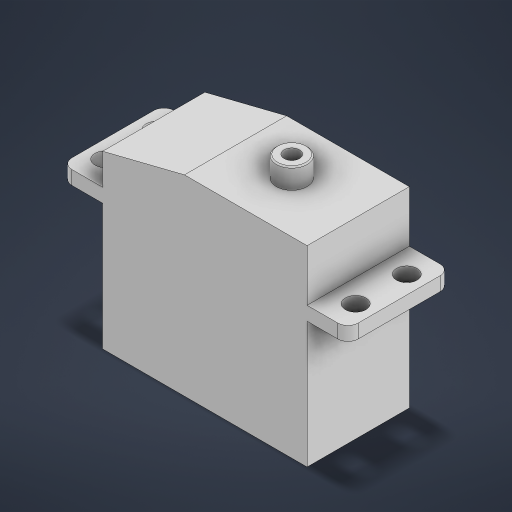
# Autodesk Inventor part: INJORA 35KG Digital Servo
Saved by Autodesk Inventor 2024 (Build 280153000, 153)
## iProperties
Created: 2024-01-29
Part Number: INJORA 35KG Digital Servo
Material: Generic
Document SubType Name: Modeling
Designer: avsar
Density: 1 g/cm^3
Appearance: Default
Author: avsar
Autodesk Inventor part; units mm, degrees
ref_plane "YZ Plane" through (0, 0, 0) normal (1, 0, 0) x (0, 1, 0)
ref_plane "XZ Plane" through (0, 0, 0) normal (0, 1, 0) x (-1, 0, 0)
ref_plane "XY Plane" through (0, 0, 0) normal (0, 0, 1) x (1, 0, 0)
sketch "Sketch1" plane through (0, 0, 0) normal (0, 1, 0) x (-1, 0, 0)
  line L0 (20, 10) -> (-20, 10)
  line L1 (-20, 10) -> (-20, -10)
  line L2 (-20, -10) -> (20, -10)
  line L3 (20, -10) -> (20, 10)
  line L4 (20, 10) -> (-20, -10) construction
  line L5 (-20, 10) -> (20, -10) construction
  point P0 (0, 0)
  dimension "d0" = 40
  dimension "d1" = 20
  constraints: 12 end point, 2 midpoint, 2 parallel, 1 horizontal, 1 perpendicular
  measures "d0" distance of L2.end L1.end
  measures "d1" distance of L1.end L0.end
extrude "Extrusion1" add sketch "Sketch1" along normal blind 37.5
ref_plane "Work Plane1" through (0, 24.7, 0) normal (0, -1, 0) x (1, 0, 0)
sketch "Sketch2" plane through (0, 24.7, 0) normal (0, -1, 0) x (1, 0, 0)
  line L0 (-28, 10) -> (28, 10)
  line L1 (28, 10) -> (28, -10)
  line L2 (28, -10) -> (-28, -10)
  line L3 (-28, -10) -> (-28, 10)
  line L4 (-28, 10) -> (28, -10) construction
  line L5 (28, 10) -> (-28, -10) construction
  point P0 (0, 0)
  dimension "d5" = 56
  dimension "d6" = 20
  constraints: 12 end point, 2 midpoint, 2 parallel, 1 horizontal, 1 perpendicular
  measures "d5" distance of L1.end L2.end
  measures "d6" distance of L0.end L1.end
extrude "Extrusion2" add sketch "Sketch2" against normal blind 2.7
sketch "Sketch3" plane through (0, 27.4, 0) normal (0, 1, 0) x (1, 0, 0)
  circle A0 centre (-24.5, -5) radius 2
  line L0 (-28, 10) -> (-28, -10) construction
  line L1 (-28, 0) -> (28, 0) construction
  line L2 (28, 10) -> (28, -10) construction
  line L3 (-20, -10) -> (20, -10) projected
  line L4 (0, -10) -> (0, 10) construction
  line L5 (20, 10) -> (-20, 10) projected
  circle A1 centre (-24.5, 5) radius 2
  circle A2 centre (24.5, -5) radius 2
  circle A3 centre (24.5, 5) radius 2
  point P0 (0, 0)
  dimension "d9" = 4
  dimension "d10" = 5
  dimension "d11" = 24.5
  constraints: 4 centre point, 4 end point, 4 midpoint, 3 symmetric about line, 3 other
  measures "d9" diameter of A0
  measures "d10" vertical distance of A0.centre point (0, 0)
  measures "d11" horizontal distance of point (0, 0) A0.centre
extrude "Extrusion3" cut sketch "Sketch3" against normal up to surface (2.7 mm away)
sketch "Sketch4" plane through (0, 37.5, 0) normal (0, 1, 0) x (1, 0, 0)
  circle A0 centre (7, 0) radius 3
  line L0 (20, -10) -> (20, 10) projected
  point P0 (0, 0)
  dimension "d14" = 6
  dimension "d15" = 13
  constraints: 1 centre point, 1 horizontal alignment
  measures "d14" diameter of A0
  measures "d15" distance from line of L0 A0.centre
extrude "Extrusion4" add sketch "Sketch4" along normal blind 4
fillet "Fillet1" radius 2 4 edges at (-28, 26.05, 10) (28, 26.05, 10) (28, 26.05, -10) (-28, 26.05, -10)
chamfer "Chamfer1" distance 16 distance2 4 1 edges at (-20, 37.5, 0) measured on face at (-19.5, 37.5, 0)
sketch "Sketch5" plane through (7, 41.5, 0) normal (0, 1, 0) x (1, 0, 0)
  circle A0 centre (0, 0) radius 1.5
  circle A1 centre (0, 0) radius 3 construction
  point P0 (-7, 0)
  dimension "d22" = 3
  constraints: 1 centre point, 1 concentric
  measures "d22" diameter of A0
extrude "Extrusion5" cut sketch "Sketch5" against normal blind 4
chamfer "Chamfer2" distance 0.25 angle 45 1 edges at (4, 41.5, 0)
body "Solid1"
